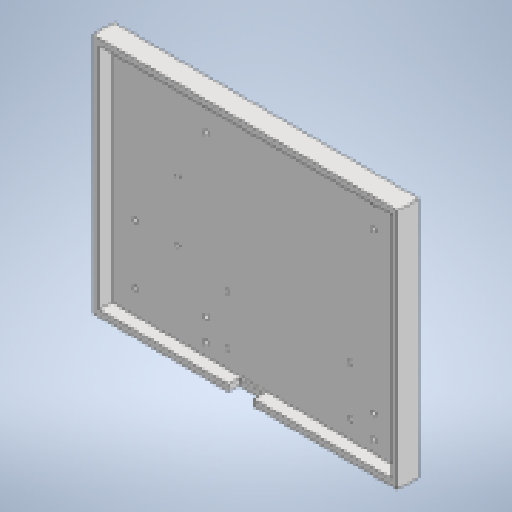
# Autodesk Inventor part: support
Saved by Autodesk Inventor 2024 (Build 280153000, 153)
## iProperties
Created: 2024-03-12
Part Number: support
Material: Générique
Document SubType Name: Modeling
Designer: phaly
Density: 1 g/cm^3
Appearance: Par défaut
Author: phaly
Autodesk Inventor part; units mm, degrees
ref_plane "YZ Plane" through (0, 0, 0) normal (1, 0, 0) x (0, 1, 0)
ref_plane "XZ Plane" through (0, 0, 0) normal (0, 1, 0) x (-1, 0, 0)
ref_plane "XY Plane" through (0, 0, 0) normal (0, 0, 1) x (1, 0, 0)
sketch "Esquisse1" plane through (0, 0, 0) normal (0, 0, 1) x (1, 0, 0)
  line L0 (0, 114) -> (144, 114)
  line L1 (144, 114) -> (144, 0)
  line L2 (144, 0) -> (0, 0)
  line L3 (0, 0) -> (0, 114)
  line L4 (3, 111) -> (141, 111)
  line L5 (141, 111) -> (141, 3)
  line L6 (141, 3) -> (3, 3)
  line L7 (3, 3) -> (3, 111)
  line L8 (0, -22.8) -> (0, 136.8) projected
  line L9 (-28.8, 0) -> (172.8, 0) projected
  point P0 (0, 0)
  dimension "d0" = 114
  dimension "d1" = 144
  dimension "d2" = 3
  dimension "d3" = 3
  dimension "d4" = 3
  dimension "d5" = 3
  constraints: 16 end point, 4 parallel, 2 collinear, 2 horizontal, 2 perpendicular
  measures "d0" distance of L2.end L0.start
  measures "d1" distance of L0.start L0.end
  measures "d2" distance between parallel lines of L0 L4
  measures "d3" distance between parallel lines of L2 L6
  measures "d4" distance between parallel lines of L3 L7
  measures "d5" distance between parallel lines of L1 L5
extrude "Extrusion1" add sketch "Esquisse1" along normal blind 10
sketch "Esquisse2" plane through (0, 0, 0) normal (0, 0, -1) x (-1, 0, 0)
  line L0 (0, 114) -> (-144, 114)
  line L1 (-144, 114) -> (-144, 0)
  line L2 (-144, 0) -> (0, 0)
  line L3 (0, 0) -> (0, 114)
  line L4 (0, 114) -> (0, 0) projected
  line L5 (-144, 114) -> (0, 114) projected
  line L6 (0, 0) -> (-144, 0) projected
  line L7 (-144, 0) -> (-144, 114) projected
  constraints: 8 end point, 4 collinear, 2 parallel, 1 horizontal, 1 perpendicular
extrude "Extrusion2" add sketch "Esquisse2" against normal blind 4
sketch "Esquisse7" plane through (0, 0, 0) normal (0, 0, -1) x (-1, 0, 0)
  arc A0 (-119, 10) -> (-117, 8) centre (-117, 10) ccw projected
  line L0 (-119, 10) -> (-119, 36) projected
  arc A1 (-117, 38) -> (-119, 36) centre (-117, 36) ccw projected
  line L1 (-117, 38) -> (-56, 38) projected
  arc A2 (-54, 36) -> (-56, 38) centre (-56, 36) ccw projected
  line L2 (-54, 36) -> (-54, 10) projected
  arc A3 (-56, 8) -> (-54, 10) centre (-56, 10) ccw projected
  line L3 (-56, 8) -> (-117, 8) projected
  line L4 (-111, 9) -> (-61, 9) projected
  line L5 (-61, 9) -> (-61, 14) projected
  line L6 (-61, 14) -> (-111, 14) projected
  line L7 (-111, 14) -> (-111, 9) projected
  circle A4 centre (-115.5, 34.5) radius 1.75 projected
  circle A5 centre (-57.5, 34.5) radius 1.75 projected
  circle A6 centre (-57.5, 11.5) radius 1.75 projected
  circle A7 centre (-115.5, 11.5) radius 1.75 projected
  circle A8 centre (-34, 70) radius 1 projected
  circle A9 centre (-34, 42) radius 1 projected
  line L8 (-42, 6) -> (-24.5, 6) projected
  line L9 (-42, 78) -> (-42, 6) projected
  line L10 (-24.5, 78) -> (-42, 78) projected
  line L11 (-24.5, 6) -> (-24.5, 78) projected
  circle A10 centre (-14, 42) radius 1 projected
  circle A11 centre (-14, 14) radius 1 projected
  line L12 (-23, 6) -> (-6, 6) projected
  line L13 (-23, 78) -> (-23, 6) projected
  line L14 (-6, 78) -> (-23, 78) projected
  line L15 (-6, 6) -> (-6, 78) projected
  point P0 (0, 0)
  constraints: 8 coincident
hole "Perçage1" at (57.5, 11.5, 0) at (57.5, 34.5, 0) at (115.5, 11.5, 0) at (115.5, 34.5, 0) at (14, 42, 0) at (34, 42, 0) at (34, 70, 0) at (14, 14, 0) direction (0, 0, 1) diameter 2 end through all
sketch "Esquisse8" plane through (0, 0, 0) normal (0, -1, 0) x (1, 0, 0)
  line L0 (66.5, 8) -> (73.5, 8) projected
  line L1 (73.5, 8) -> (73.5, 12) projected
  line L2 (66.5, 12) -> (73.5, 12) projected
  line L3 (66.5, 8) -> (66.5, 12) projected
  line L4 (76, 5) -> (64, 5)
  line L5 (64, 5) -> (64, 10)
  line L6 (64, 10) -> (76, 10)
  line L7 (76, 10) -> (76, 5)
  line L8 (0, 10) -> (144, 10) projected
  line L9 (70, -1.8749) -> (70, 11.0144)
  point P0 (0, 0)
  dimension "d43" = 12
  dimension "d44" = 3.5
  dimension "d45" = 5
  constraints: 10 end point, 2 parallel, 1 collinear, 1 horizontal, 1 perpendicular, 1 vertical, 1 other
  measures "d43" distance of L4.start L4.end
  measures "d44" distance between parallel lines of L1 L9
  measures "d45" distance of L6.end L4.start
extrude "Extrusion6" cut sketch "Esquisse8" against normal blind 10 contours L3 L6 L9 L0 | L0 L9 L4 L5 L6 L3 | L9 L6 L1 L0 | L0 L1 L6 L7 L4 L9
sketch "Esquisse11" plane through (0, 0, 0) normal (0, 0, -1) x (-1, 0, 0)
  line L0 (0, 0) -> (-144, 0) projected
  line L1 (-144, 114) -> (0, 114) projected
  line L2 (-144, 0) -> (-144, 114) projected
  point P0 (-47.5, 105.5)
  point P1 (-126.5, 105.5)
  point P2 (-126.5, 8.5)
  point P3 (-47.5, 8.5)
  point P4 (-47.5, 94.5)
  point P5 (-47.5, 19.5)
  point P6 (-126.5, 19.5)
  point P7 (-126.5, 94.5)
  dimension "d54" = 79
  dimension "d55" = 79
  dimension "d56" = 97
  dimension "d57" = 97
  dimension "d58" = 8.5
  dimension "d59" = 8.5
  dimension "d60" = 8.5
  dimension "d68" = 17.5
  dimension "d69" = 79
  dimension "d70" = 79
  dimension "d71" = 75
  dimension "d72" = 75
  dimension "d73" = 11
  dimension "d74" = 11
  dimension "d75" = 17.5
  dimension "d76" = 19.5
  measures "d54" distance of point (-126.5, 105.5) point (-47.5, 105.5)
  measures "d55" distance of point (-126.5, 8.5) point (-47.5, 8.5)
  measures "d56" distance of point (-47.5, 8.5) point (-47.5, 105.5)
  measures "d57" distance of point (-126.5, 8.5) point (-126.5, 105.5)
  measures "d58" distance from line of L0 point (-47.5, 8.5)
  measures "d59" distance from line of L0 point (-126.5, 8.5)
  measures "d60" distance from line of L1 point (-47.5, 105.5)
  measures "d68" distance from line of L2 point (-126.5, 8.5)
  measures "d69" distance of point (-126.5, 94.5) point (-47.5, 94.5)
  measures "d70" distance of point (-126.5, 19.5) point (-47.5, 19.5)
  measures "d71" distance of point (-126.5, 19.5) point (-126.5, 94.5)
  measures "d72" distance of point (-47.5, 19.5) point (-47.5, 94.5)
  measures "d73" distance of point (-47.5, 8.5) point (-47.5, 19.5)
  measures "d74" distance of point (-126.5, 8.5) point (-126.5, 19.5)
  measures "d75" distance from line of L2 point (-126.5, 19.5)
  measures "d76" distance from line of L1 point (-47.5, 94.5)
hole "Perçage2" at (47.5, 105.5, 0) at (126.5, 105.5, 0) at (126.5, 8.5, 0) at (47.5, 8.5, 0) at (47.5, 94.5, 0) at (47.5, 19.5, 0) at (126.5, 94.5, 0) at (126.5, 19.5, 0) direction (0, 0, 1) diameter 2.5 end through all
equation "\"d3\" = d2"
equation "\"d4\" = d3"
equation "\"d5\" = d4"
equation "\"d55\" = d54"
equation "\"d57\" = d56"
equation "\"d59\" = d58"
equation "\"d60\" = d58"
equation "\"d69\" = d54"
equation "\"d70\" = d55"
equation "\"d72\" = d71"
equation "\"d74\" = d73"
equation "\"d75\" = d68"
